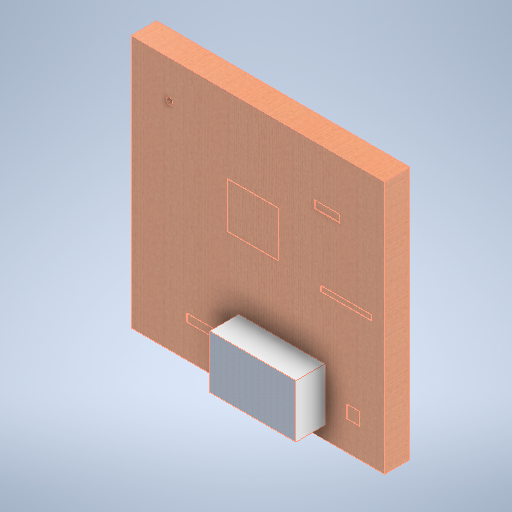
# Autodesk Inventor part: Base
Saved by Autodesk Inventor 2025.3 (Build 293356000, 356)
## iProperties
Created: 2026-03-11
Part Number: Base
Material: Generic
Document SubType Name: Modeling
Designer: logien
Density: 1 g/cm^3
Appearance: Red Oak - Natural Low Gloss
Author: logien
Autodesk Inventor part; units mm, degrees
sketch "Sketch1" plane through (0, 0, 0) normal (0, 0, 1) x (1, 0, 0)
  line L0 (0, 0) -> (1000, 0)
  line L1 (1000, 0) -> (1000, 1000)
  line L2 (1000, 1000) -> (0, 1000)
  line L3 (0, 1000) -> (0, 0)
  dimension "d0" = 1000
  dimension "d1" = 1000
  constraints: 8 end point, 2 parallel, 1 horizontal, 1 perpendicular
  measures "d0" distance of L1.end L2.end
  measures "d1" distance of L2.end L0.start
extrude "Extrusion1" add sketch "Sketch1" along normal blind 100
sketch "Sketch8" plane through (0, 0, 100) normal (0, 0, 1) x (1, 0, 0)
  line L0 (1000, 1000) -> (0, 1000) projected
  line L1 (0, 1000) -> (150, 1000)
  line L2 (150, 1000) -> (150, 850)
  circle A0 centre (150, 850) radius 12.5
  point P0 (0, 0)
  dimension "d30" = 150
  dimension "d31" = 150
  dimension "d32" = 25
  constraints: 4 end point, 1 centre point, 1 coincident, 1 perpendicular, 1 point on line
  measures "d30" distance of L0.end L1.end
  measures "d31" distance of L1.end L2.end
  measures "d32" diameter of A0
extrude "Extrusion4" cut sketch "Sketch8" against normal blind 100
sketch "Sketch9" plane through (0, 0, 100) normal (0, 0, 1) x (1, 0, 0)
  line L0 (425, 260) -> (765, 260)
  line L1 (765, 260) -> (765, 50)
  line L2 (765, 50) -> (425, 50)
  line L3 (425, 50) -> (425, 260)
  line L4 (0, 0) -> (1000, 0) projected
  line L5 (0, 1000) -> (0, 0) projected
  dimension "d35" = 210
  dimension "d36" = 340
  dimension "d37" = 50
  constraints: 8 end point, 2 parallel, 1 horizontal, 1 perpendicular
  measures "d35" distance of L2.end L0.start
  measures "d36" distance of L1.end L2.end
  measures "d37" distance between parallel lines of L4 L2
extrude "Extrusion5" add sketch "Sketch9" along normal blind 115
ref_plane "Work Plane6" through (1000, 0, 0) normal (1, 0, 0) x (0, 0, -1)
ref_plane "Work Plane7" through (0, 775, 0) normal (0, 1, 0) x (1, 0, 0)
sketch "Sketch12" plane through (0, 0, 100) normal (0, 0, 1) x (1, 0, 0)
  line L0 (0, 0) -> (1000, 0) projected
  line L1 (877, 141) -> (742, 141) construction
  line L2 (877, 141) -> (877, 166) construction
  line L3 (902, 166) -> (902, 116)
  line L4 (902, 116) -> (852, 116)
  line L5 (852, 116) -> (852, 166)
  line L6 (852, 166) -> (902, 166)
  dimension "d58" = 25
  dimension "d59" = 50
  dimension "d60" = 50
  dimension "d63" = 25
  dimension "d64" = 25
  constraints: 12 end point, 3 perpendicular, 2 vertical, 1 horizontal
  measures "d58" distance of L1.start L2.end
  measures "d59" distance of L3.start L3.end
  measures "d60" distance of L3.end L4.end
  measures "d63" distance from line of L3 L1.start
  measures "d64" distance from line of L4 L1.start
extrude "Extrusion8" add sketch "Sketch12" along normal blind 0.5
ref_plane "Work Plane8" through (0, 237, 0) normal (0, -1, 0) x (1, 0, 0)
sketch "Sketch13" plane through (0, 0, 100) normal (0, 0, 1) x (1, 0, 0)
  line L0 (425, 260) -> (425, 50) projected
  line L1 (425, 155) -> (395, 155)
  line L2 (395, 155) -> (395, 160)
  line L3 (395, 160) -> (220, 160)
  line L4 (220, 160) -> (220, 130)
  line L5 (220, 130) -> (395, 130)
  line L6 (395, 130) -> (395, 155)
  line L7 (425, 50) -> (164, 50)
  point P0 (0, 0)
  dimension "d67" = 30
  dimension "d68" = 5
  dimension "d69" = 175
  dimension "d73" = 80
  constraints: 14 end point, 4 perpendicular, 3 horizontal, 1 midpoint
  measures "d67" distance of L1.start L1.end
  measures "d68" distance of L1.end L2.end
  measures "d69" distance of L2.end L3.end
  measures "d73" distance between parallel lines of L7 L5
extrude "Extrusion9" cut sketch "Sketch13" against normal blind 1
sketch "Sketch14" plane through (0, 0, 100) normal (0, 0, 1) x (1, 0, 0)
  line L0 (580, 520) -> (380, 520)
  line L1 (380, 520) -> (380, 700)
  line L2 (380, 700) -> (580, 700)
  line L3 (580, 700) -> (580, 520)
  line L4 (0, 1000) -> (0, 0) projected
  line L5 (1000, 1000) -> (0, 1000) projected
  point P0 (380, 610)
  dimension "d74" = 180
  dimension "d75" = 200
  dimension "d76" = 380
  dimension "d77" = 300
  constraints: 8 end point, 2 parallel, 1 horizontal, 1 midpoint, 1 perpendicular
  measures "d74" distance of L0.end L1.end
  measures "d75" distance of L1.end L2.end
  measures "d76" distance from line of L4 point (380, 610)
  measures "d77" distance between parallel lines of L5 L2
extrude "Extrusion10" cut sketch "Sketch14" against normal blind 1
sketch "Sketch16" plane through (0, 0, 100) normal (0, 0, 1) x (1, 0, 0)
  line L0 (722.7051, 770) -> (822.7051, 770)
  line L1 (822.7051, 770) -> (822.7051, 800)
  line L2 (822.7051, 800) -> (722.7051, 800)
  line L3 (722.7051, 800) -> (722.7051, 770)
  line L4 (1000, 1000) -> (0, 1000) projected
  point P0 (0, 0)
  dimension "d86" = 100
  dimension "d87" = 30
  dimension "d90" = 200
  constraints: 8 end point, 2 parallel, 1 horizontal, 1 perpendicular
  measures "d86" distance of L0.start L0.end
  measures "d87" distance of L0.end L1.end
  measures "d90" distance between parallel lines of L4 L2
extrude "Extrusion12" cut sketch "Sketch16" against normal blind 3
sketch "Sketch18" plane through (0, 0, 100) normal (0, 0, 1) x (1, 0, 0)
  line L0 (950, 500) -> (750, 500)
  line L1 (750, 500) -> (750, 520)
  line L2 (750, 520) -> (950, 520)
  line L3 (950, 520) -> (950, 500)
  line L4 (1000, 0) -> (1000, 1000) projected
  line L5 (0, 0) -> (1000, 0) projected
  dimension "d93" = 20
  dimension "d94" = 50
  dimension "d95" = 500
  dimension "d96" = 200
  constraints: 8 end point, 2 parallel, 1 horizontal, 1 perpendicular
  measures "d93" distance of L0.end L1.end
  measures "d94" distance between parallel lines of L4 L3
  measures "d95" distance between parallel lines of L5 L0
  measures "d96" distance of L1.end L2.end
extrude "Extrusion14" add sketch "Sketch18" along normal blind 1
body "Solid1"
